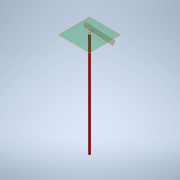
# Autodesk Inventor part: redWire
Saved by Autodesk Inventor 2022 (Build 260153000, 153)
## iProperties
Created: 2022-02-03
Part Number: redWire
Material: Generic
Document SubType Name: Modeling
Designer: tecware
Density: 1 g/cm^3
Appearance: Default
Author: tecware
Autodesk Inventor part; units mm, degrees
ref_plane "YZ Plane" through (0, 0, 0) normal (1, 0, 0) x (0, 1, 0)
ref_plane "XZ Plane" through (0, 0, 0) normal (0, 1, 0) x (-1, 0, 0)
ref_plane "XY Plane" through (0, 0, 0) normal (0, 0, 1) x (1, 0, 0)
ref_plane "Work Plane2" through (3.5859, 0, -0.978) normal (0, -1, 0) x (1, 0, 0)
sketch "Sketch2" plane through (3.5859, 0, -0.978) normal (0, -1, 0) x (1, 0, 0)
  circle A0 centre (0, 0) radius 0.675
  point P0 (-3.5859, 0.978)
  dimension "d3" = 1.35
  constraints: 1 centre point
  measures "d3" diameter of A0
extrude "Extrusion2" add sketch "Sketch2" along normal blind 71.25
ref_plane "Work Plane1" through (3.5859, 3, -0.978) normal (0, 1, 0) x (1, 0, 0)
sketch "Sketch3" plane through (3.5859, 0, -0.978) normal (0, 1, 0) x (1, 0, 0)
  circle A0 centre (0, 0) radius 0.315
  point P0 (-3.5859, -0.978)
  dimension "d7" = 0.63
  constraints: 1 centre point
  measures "d7" diameter of A0
extrude "Extrusion3" add sketch "Sketch3" along normal blind 1.5
ref_plane "Work Plane3" through (5.9115, 2.4915, -1.92) normal (0.4330127, 0.8660254, -0.25) x (0.5, 0, 0.8660254)
sketch "Sketch5" plane through (5.9115, 2.4915, -1.92) normal (0.4330127, 0.8660254, -0.25) x (0.5, 0, 0.8660254)
  circle A0 centre (-0.4635, -1.064) radius 0.315
  point P0 (-1.293, -4.0192)
  dimension "d11" = 0.63
  constraints: 1 centre point
  measures "d11" diameter of A0
loft "Loft1" add profiles "Sketch5" section 1 edges at (3.2709, 1.5, -0.978)
body "Solid1"
